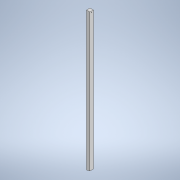
# Autodesk Inventor part: Stand Leg
Saved by Autodesk Inventor 2022 (Build 260153000, 153)
## iProperties
Created: 2023-09-19
Part Number: Stand Leg
Material: Generic
Document SubType Name: Modeling
Designer: fouad
Density: 1 g/cm^3
Appearance: Default
Author: fouad
Autodesk Inventor part; units mm, degrees
ref_plane "YZ Plane" through (0, 0, 0) normal (1, 0, 0) x (0, 1, 0)
ref_plane "XZ Plane" through (0, 0, 0) normal (0, 1, 0) x (-1, 0, 0)
ref_plane "XY Plane" through (0, 0, 0) normal (0, 0, 1) x (1, 0, 0)
sketch "Sketch1" plane through (0, 0, 0) normal (0, 1, 0) x (-1, 0, 0)
  line L0 (2.5, 2.5) -> (-2.5, 2.5)
  line L1 (-2.5, 2.5) -> (-2.5, -2.5)
  line L2 (-2.5, -2.5) -> (2.5, -2.5)
  line L3 (2.5, -2.5) -> (2.5, 2.5)
  point P0 (0, 0)
  dimension "d0" = 5
  dimension "d1" = 5
  dimension "d2" = 2.5
  dimension "d3" = 2.5
  constraints: 8 end point, 2 parallel, 1 horizontal, 1 perpendicular
  measures "d0" distance of L2.end L1.end
  measures "d1" distance of L1.end L0.end
  measures "d2" distance from line of point (0, 0) L2
  measures "d3" distance from line of point (0, 0) L1
extrude "Extrusion1" add sketch "Sketch1" along normal blind 200
sketch "Sketch3" plane through (2.5, 200, 2.5) normal (1, 0, 0) x (0, 0, -1)
  circle A0 centre (2.5, -2) radius 0.375
  line L0 (0, 0) -> (5, 0) projected
  line L1 (5, -200) -> (5, 0) projected
  point P0 (2.5, -200)
  point P1 (5, -198.6603)
  dimension "d9" = 0.75
  dimension "d10" = 2
  dimension "d11" = 2.5
  constraints: 1 centre point
  measures "d9" diameter of A0
  measures "d10" distance from line of A0.centre L0
  measures "d11" distance from line of A0.centre L1
extrude "Extrusion3" cut sketch "Sketch3" against normal blind 200
sketch "Sketch4" plane through (-2.5, 0, 2.5) normal (0, 0, 1) x (1, 0, 0)
  line L0 (5, 0) -> (0, 0) projected
  line L1 (0, 0) -> (5, 1.3397)
  line L2 (5, 0) -> (5, 200) projected
  line L3 (0, 0) -> (5.1764, 0) construction
  line L4 (5, 1.3397) -> (5, 0)
  line L5 (5, 0) -> (0, 0)
  point P0 (2.5, 0)
  dimension "d14" = 15
  constraints: 8 end point, 1 collinear, 1 equal length, 1 horizontal, 1 perpendicular, 1 point on line
  measures "d14" angle of L3 L1
extrude "Extrusion4" cut sketch "Sketch4" against normal blind 200
body "Solid1"
